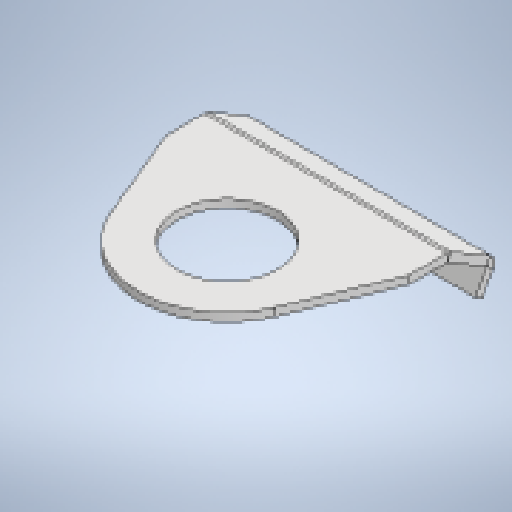
# Autodesk Inventor part: NVPH-306 front side
Saved by Autodesk Inventor 2025.1 (Build 291241020, 241B)
## iProperties
Created: 2024-12-03
Part Number: NVPH-306 front side
Material: Generic
Document SubType Name: Sheet Metal
Designer: admin
Density: 1 g/cm^3
Sheet Metal Rule: Default
Appearance: Default
Author: user
Autodesk Inventor part; units mm, degrees
ref_plane "YZ Plane" through (0, 0, 0) normal (1, 0, 0) x (0, 1, 0)
ref_plane "XZ Plane" through (0, 0, 0) normal (0, 1, 0) x (-1, 0, 0)
ref_plane "XY Plane" through (0, 0, 0) normal (0, 0, 1) x (1, 0, 0)
sketch "Sketch1" plane through (0, 0, 0) normal (0, 0, 1) x (1, 0, 0)
  line L0 (0, 0) -> (0, 234.6882)
  line L1 (-150, 234.6882) -> (150, 234.6882)
  circle A0 centre (0, 110) radius 62.5
  circle A1 centre (0, 110) radius 110
  line L2 (-150, 234.6882) -> (-150, 184.6882)
  line L3 (-150, 184.6882) -> (-101.6267, 67.9048)
  line L4 (150, 234.6882) -> (150, 184.6882)
  line L5 (150, 184.6882) -> (101.6267, 67.9048)
  dimension "d0" = 234.6882
  dimension "d1" = 300
  dimension "d2" = 125
  dimension "d4" = 50
  dimension "d17" = 45
  dimension "d18" = 220
  measures "d0" distance of L0.end L0.start
  measures "d1" distance of L1.start L1.end
  measures "d2" diameter of A0
  measures "d4" distance of L1.start L2.end
  measures "d17" angle of L5 L3
  measures "d18" diameter of A1
extrude "Plate1" add sketch "Sketch1" along normal blind 10 contours A1 L0 A0 | L0 A0 A1 | L3 L2 L1 L0 A1 | A1 L0 L1 L4 L5
sketch "Sketch3" plane through (150, 229.6882, 1.3397) normal (0, 0.5, 0.8660254) x (-1, 0, 0)
  line L0 (300, 0) -> (0, 0)
  line L1 (0, 0) -> (0, -70)
  line L2 (0, -70) -> (300, -70)
  line L3 (300, -70) -> (300, 0)
  constraints: 6 end point, 1 horizontal, 1 perpendicular, 1 vertical
edge flange "Flange2" height 70 angle 30 thickness 10 bend radius 1 thickness toward (0, 0.5, 0.8660254) relief straight relief width 10 relief depth 5 edges at (0, 234.6882, 0) wall of the first edge with corners at (-150, 229.6882, 1.3397) (150, 229.6882, 1.3397) (150, 290.31, -33.6603) (-150, 290.31, -33.6603)
bend "Bend2"
corner "Corner2"
sketch "Sketch4" plane through (150, 286.6497, -20) normal (0, 0.8660254, -0.5) x (-1, 0, 0)
  line L0 (300, 0) -> (0, 0)
  line L1 (0, 0) -> (0, -40)
  line L2 (0, -40) -> (300, -40)
  line L3 (300, -40) -> (300, 0)
  constraints: 6 end point, 1 horizontal, 1 perpendicular, 1 vertical
edge flange "Flange3" height 40 angle 90 thickness 10 bend radius 1 thickness toward (0, 0.8660254, -0.5) relief straight relief width 10 relief depth 5 edges at (0, 290.31, -33.6603) wall of the first edge with corners at (-150, 286.6497, -20) (150, 286.6497, -20) (150, 266.6497, -54.641) (-150, 266.6497, -54.641)
bend "Bend3"
corner "Corner3"
equation "\"d2\" = back_steel_circle_проходной_диаметр"
equation "\"d5\" = Thickness"
equation "\"d19\" = BendReliefWidth"
equation "\"d20\" = BendReliefDepth"
equation "\"d21\" = MinimumRemnant"
equation "\"d22\" = TransitionRadius"
equation "\"d26\" = CornerReliefSize"
equation "\"d27\" = GapSize"
equation "\"d28\" = JacobiRadiusSize"
equation "\"d29\" = BendReliefWidth"
equation "\"d30\" = BendReliefDepth"
equation "\"d31\" = MinimumRemnant"
equation "\"d32\" = TransitionRadius"
equation "\"d36\" = CornerReliefSize"
equation "\"d37\" = GapSize"
equation "\"d38\" = JacobiRadiusSize"
equation "\"BendReliefDepth\" = 0.5 * Thickness"
equation "\"back_steel_circle_проходной_диаметр\" = 125"
equation "\"Thickness\" = 10"
equation "\"BendReliefWidth\" = 10"
equation "\"MinimumRemnant\" = 20"
equation "\"TransitionRadius\" = 10"
equation "\"CornerReliefSize\" = 40"
equation "\"GapSize\" = 10"
equation "\"JacobiRadiusSize\" = 10"
body "Solid1"
